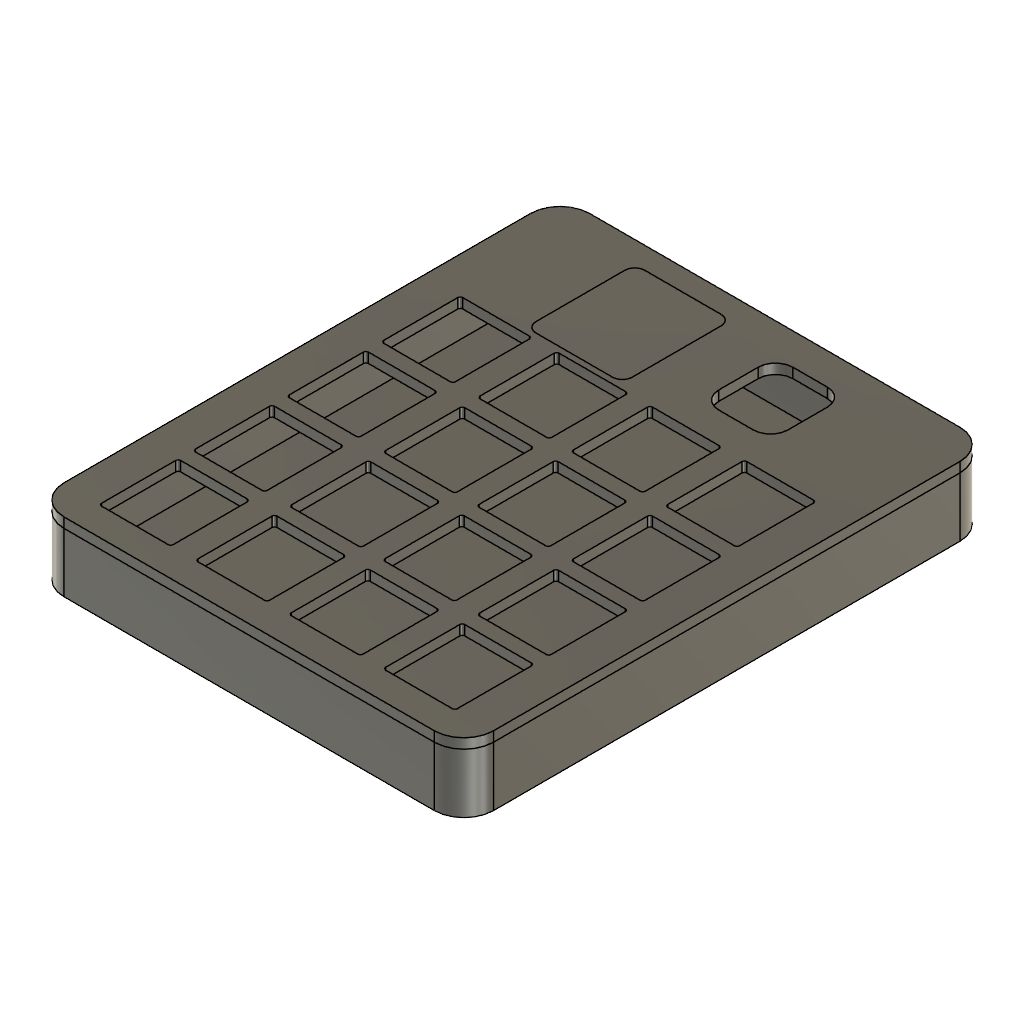
Untitled (Autodesk Fusion 360 design; units mm, degrees)
part number: 2026-09-21-00-24-33-049
Autodesk Fusion 360 part; units mm, degrees
sketch "Sketch2" plane through (0, 0, 0) normal (0, 0, 1) x (1, 0, 0)
sketch "Sketch3" plane through (0, 0, 0) normal (0, 0, 1) x (1, 0, 0)
  line L0 (0, 0) -> (80.94, 0)
  line L1 (80.94, 0) -> (80.94, 100.4)
  line L2 (80.94, 100.4) -> (0, 100.4)
  line L3 (0, 100.4) -> (0, 0)
  line L4 (3, 103.4) -> (77.94, 103.4)
  line L5 (83.94, 97.4) -> (83.94, 3)
  line L6 (77.94, -3) -> (3, -3)
  line L7 (-3, 3) -> (-3, 97.4)
  arc A0 (77.94, -3) -> (83.94, 3) centre (77.94, 3) ccw
  arc A1 (83.94, 97.4) -> (77.94, 103.4) centre (77.94, 97.4) ccw
  arc A2 (3, 103.4) -> (-3, 97.4) centre (3, 97.4) ccw
  arc A3 (-3, 3) -> (3, -3) centre (3, 3) ccw
  point P0 (82.94, -2)
  point P1 (-2, -2)
  point P2 (-3, 103.4)
  point P3 (83.94, 103.4)
  dimension "d5" = 80.94
  dimension "d6" = 100.4
  dimension "d26" = 86.94
  dimension "d27" = 6
  constraint horizontal L0
  constraint vertical L1
  constraint horizontal L2
  constraint vertical L3
  constraint coincident L0.start L3.end
  constraint perpendicular L1 L4
  constraint perpendicular L0 L5
  constraint perpendicular L5 L6
  constraint perpendicular L4 L7
  constraint tangent L5 A0
  constraint tangent L6 A0
  constraint coincident P3 L4
  constraint coincident P3 L5
  constraint tangent L4 A1
  constraint tangent L5 A1
  constraint equal A0 A1
  constraint coincident P2 L4
  constraint coincident P2 L7
  constraint tangent L4 A2
  constraint tangent L7 A2
  constraint equal A0 A2
  constraint tangent L6 A3
  constraint tangent L7 A3
  constraint equal A0 A3
  measures "d5" distance of L0.start L0.end
  measures "d6" distance of L0.start L2.end
  measures "d26" distance of P2 P3
  measures "d27" radius of A0
extrude "Extrude9" add sketch "Sketch3" along normal blind 2 contours L0 L1 L2 L3 | L4 L5 L6 L7 A0 A1 A2 A3 makes body 1
extrude "Extrude10" add sketch "Sketch3" along normal blind 12 bodies 1
sketch "Sketch4" plane through (0, 0, 12) normal (0, 0, 1) x (-1, 0, 0)
  line L0 (0, 0) -> (0, -100.4)
  line L1 (0, -100.4) -> (-80.94, -100.4)
  line L2 (-80.94, -100.4) -> (-80.94, 0)
  line L3 (-80.94, 0) -> (0, 0)
  arc A0 (-3, -103.4) -> (3, -97.4) centre (-3, -97.4) ccw
  line L4 (3, -97.4) -> (3, -3)
  arc A1 (3, -3) -> (-3, 3) centre (-3, -3) ccw
  line L5 (-3, 3) -> (-77.94, 3)
  arc A2 (-77.94, 3) -> (-83.94, -3) centre (-77.94, -3) ccw
  line L6 (-83.94, -3) -> (-83.94, -97.4)
  arc A3 (-83.94, -97.4) -> (-77.94, -103.4) centre (-77.94, -97.4) ccw
  line L7 (-77.94, -103.4) -> (-3, -103.4)
  line L8 (0, 0) -> (-80.94, 0)
  line L9 (-80.94, 0) -> (-80.94, -100.4)
  line L10 (-80.94, -100.4) -> (0, -100.4)
  line L11 (0, -100.4) -> (0, 0)
  line L12 (-4.9, -75.8) -> (-18.4, -75.8)
  line L13 (-18.9, -75.3) -> (-18.9, -60.3)
  line L14 (-18.4, -59.8) -> (-4.9, -59.8)
  line L15 (-4.4, -60.3) -> (-4.4, -75.3)
  line L16 (-38.4, -75.3) -> (-38.4, -60.3)
  line L17 (-37.9, -59.8) -> (-24.4, -59.8)
  line L18 (-23.9, -60.3) -> (-23.9, -75.3)
  line L19 (-24.4, -75.8) -> (-37.9, -75.8)
  line L20 (-57.3, -75.3) -> (-57.3, -60.3)
  line L21 (-56.8, -59.8) -> (-43.3, -59.8)
  line L22 (-42.8, -60.3) -> (-42.8, -75.3)
  line L23 (-43.3, -75.8) -> (-56.8, -75.8)
  line L24 (-76.4, -75.3) -> (-76.4, -60.3)
  line L25 (-75.9, -59.8) -> (-62.4, -59.8)
  line L26 (-61.9, -60.3) -> (-61.9, -75.3)
  line L27 (-62.4, -75.8) -> (-75.9, -75.8)
  line L28 (-4.4, -41.2) -> (-4.4, -56.2)
  line L29 (-18.4, -40.7) -> (-4.9, -40.7)
  line L30 (-18.9, -56.2) -> (-18.9, -41.2)
  line L31 (-4.9, -56.7) -> (-18.4, -56.7)
  line L32 (-23.9, -41.2) -> (-23.9, -56.2)
  line L33 (-24.4, -56.7) -> (-37.9, -56.7)
  line L34 (-38.4, -56.2) -> (-38.4, -41.2)
  line L35 (-37.9, -40.7) -> (-24.4, -40.7)
  line L36 (-42.8, -41.2) -> (-42.8, -56.2)
  line L37 (-56.8, -40.7) -> (-43.3, -40.7)
  line L38 (-57.3, -56.2) -> (-57.3, -41.2)
  line L39 (-43.3, -56.7) -> (-56.8, -56.7)
  line L40 (-62.4, -56.7) -> (-75.9, -56.7)
  line L41 (-61.9, -41.2) -> (-61.9, -56.2)
  line L42 (-75.9, -40.7) -> (-62.4, -40.7)
  line L43 (-76.4, -56.2) -> (-76.4, -41.2)
  line L44 (-4.4, -22.2) -> (-4.4, -37.2)
  line L45 (-18.4, -21.7) -> (-4.9, -21.7)
  line L46 (-18.9, -37.2) -> (-18.9, -22.2)
  line L47 (-4.9, -37.7) -> (-18.4, -37.7)
  line L48 (-23.9, -22.2) -> (-23.9, -37.2)
  line L49 (-24.4, -37.7) -> (-37.9, -37.7)
  line L50 (-38.4, -37.2) -> (-38.4, -22.2)
  line L51 (-37.9, -21.7) -> (-24.4, -21.7)
  line L52 (-42.8, -22.2) -> (-42.8, -37.2)
  line L53 (-56.8, -21.7) -> (-43.3, -21.7)
  line L54 (-57.3, -37.2) -> (-57.3, -22.2)
  line L55 (-43.3, -37.7) -> (-56.8, -37.7)
  line L56 (-62.4, -37.7) -> (-75.9, -37.7)
  line L57 (-61.9, -22.2) -> (-61.9, -37.2)
  line L58 (-75.9, -21.7) -> (-62.4, -21.7)
  line L59 (-76.4, -37.2) -> (-76.4, -22.2)
  line L60 (-4.4, -3.2) -> (-4.4, -18.2)
  line L61 (-18.4, -2.7) -> (-4.9, -2.7)
  line L62 (-18.9, -18.2) -> (-18.9, -3.2)
  line L63 (-4.9, -18.7) -> (-18.4, -18.7)
  line L64 (-23.9, -3.2) -> (-23.9, -18.2)
  line L65 (-24.4, -18.7) -> (-37.9, -18.7)
  line L66 (-38.4, -18.2) -> (-38.4, -3.2)
  line L67 (-37.9, -2.7) -> (-24.4, -2.7)
  line L68 (-42.8, -3.2) -> (-42.8, -18.2)
  line L69 (-56.8, -2.7) -> (-43.3, -2.7)
  line L70 (-57.3, -18.2) -> (-57.3, -3.2)
  line L71 (-43.3, -18.7) -> (-56.8, -18.7)
  line L72 (-62.4, -18.7) -> (-75.9, -18.7)
  line L73 (-61.9, -3.2) -> (-61.9, -18.2)
  line L74 (-75.9, -2.7) -> (-62.4, -2.7)
  line L75 (-76.4, -18.2) -> (-76.4, -3.2)
  line L76 (-50.5, -97) -> (-57.5, -97)
  line L77 (-61, -93.5) -> (-61, -85.5)
  line L78 (-57.5, -82) -> (-50.5, -82)
  line L79 (-47, -85.5) -> (-47, -93.5)
  arc A4 (-18.9, -75.3) -> (-18.4, -75.8) centre (-18.4, -75.3) ccw
  arc A5 (-18.4, -59.8) -> (-18.9, -60.3) centre (-18.4, -60.3) ccw
  arc A6 (-4.4, -60.3) -> (-4.9, -59.8) centre (-4.9, -60.3) ccw
  arc A7 (-4.9, -75.8) -> (-4.4, -75.3) centre (-4.9, -75.3) ccw
  arc A8 (-24.4, -75.8) -> (-23.9, -75.3) centre (-24.4, -75.3) ccw
  arc A9 (-38.4, -75.3) -> (-37.9, -75.8) centre (-37.9, -75.3) ccw
  arc A10 (-37.9, -59.8) -> (-38.4, -60.3) centre (-37.9, -60.3) ccw
  arc A11 (-23.9, -60.3) -> (-24.4, -59.8) centre (-24.4, -60.3) ccw
  arc A12 (-42.8, -60.3) -> (-43.3, -59.8) centre (-43.3, -60.3) ccw
  arc A13 (-56.8, -59.8) -> (-57.3, -60.3) centre (-56.8, -60.3) ccw
  arc A14 (-57.3, -75.3) -> (-56.8, -75.8) centre (-56.8, -75.3) ccw
  arc A15 (-43.3, -75.8) -> (-42.8, -75.3) centre (-43.3, -75.3) ccw
  arc A16 (-62.4, -75.8) -> (-61.9, -75.3) centre (-62.4, -75.3) ccw
  arc A17 (-61.9, -60.3) -> (-62.4, -59.8) centre (-62.4, -60.3) ccw
  arc A18 (-75.9, -59.8) -> (-76.4, -60.3) centre (-75.9, -60.3) ccw
  arc A19 (-76.4, -75.3) -> (-75.9, -75.8) centre (-75.9, -75.3) ccw
  arc A20 (-76.4, -56.2) -> (-75.9, -56.7) centre (-75.9, -56.2) ccw
  arc A21 (-75.9, -40.7) -> (-76.4, -41.2) centre (-75.9, -41.2) ccw
  arc A22 (-61.9, -41.2) -> (-62.4, -40.7) centre (-62.4, -41.2) ccw
  arc A23 (-62.4, -56.7) -> (-61.9, -56.2) centre (-62.4, -56.2) ccw
  arc A24 (-57.3, -56.2) -> (-56.8, -56.7) centre (-56.8, -56.2) ccw
  arc A25 (-43.3, -56.7) -> (-42.8, -56.2) centre (-43.3, -56.2) ccw
  arc A26 (-42.8, -41.2) -> (-43.3, -40.7) centre (-43.3, -41.2) ccw
  arc A27 (-56.8, -40.7) -> (-57.3, -41.2) centre (-56.8, -41.2) ccw
  arc A28 (-37.9, -40.7) -> (-38.4, -41.2) centre (-37.9, -41.2) ccw
  arc A29 (-38.4, -56.2) -> (-37.9, -56.7) centre (-37.9, -56.2) ccw
  arc A30 (-24.4, -56.7) -> (-23.9, -56.2) centre (-24.4, -56.2) ccw
  arc A31 (-23.9, -41.2) -> (-24.4, -40.7) centre (-24.4, -41.2) ccw
  arc A32 (-18.4, -40.7) -> (-18.9, -41.2) centre (-18.4, -41.2) ccw
  arc A33 (-18.9, -56.2) -> (-18.4, -56.7) centre (-18.4, -56.2) ccw
  arc A34 (-4.9, -56.7) -> (-4.4, -56.2) centre (-4.9, -56.2) ccw
  arc A35 (-4.4, -41.2) -> (-4.9, -40.7) centre (-4.9, -41.2) ccw
  arc A36 (-4.9, -37.7) -> (-4.4, -37.2) centre (-4.9, -37.2) ccw
  arc A37 (-4.4, -22.2) -> (-4.9, -21.7) centre (-4.9, -22.2) ccw
  arc A38 (-18.4, -21.7) -> (-18.9, -22.2) centre (-18.4, -22.2) ccw
  arc A39 (-18.9, -37.2) -> (-18.4, -37.7) centre (-18.4, -37.2) ccw
  arc A40 (-24.4, -37.7) -> (-23.9, -37.2) centre (-24.4, -37.2) ccw
  arc A41 (-23.9, -22.2) -> (-24.4, -21.7) centre (-24.4, -22.2) ccw
  arc A42 (-37.9, -21.7) -> (-38.4, -22.2) centre (-37.9, -22.2) ccw
  arc A43 (-38.4, -37.2) -> (-37.9, -37.7) centre (-37.9, -37.2) ccw
  arc A44 (-43.3, -37.7) -> (-42.8, -37.2) centre (-43.3, -37.2) ccw
  arc A45 (-42.8, -22.2) -> (-43.3, -21.7) centre (-43.3, -22.2) ccw
  arc A46 (-56.8, -21.7) -> (-57.3, -22.2) centre (-56.8, -22.2) ccw
  arc A47 (-57.3, -37.2) -> (-56.8, -37.7) centre (-56.8, -37.2) ccw
  arc A48 (-62.4, -37.7) -> (-61.9, -37.2) centre (-62.4, -37.2) ccw
  arc A49 (-61.9, -22.2) -> (-62.4, -21.7) centre (-62.4, -22.2) ccw
  arc A50 (-75.9, -21.7) -> (-76.4, -22.2) centre (-75.9, -22.2) ccw
  arc A51 (-76.4, -37.2) -> (-75.9, -37.7) centre (-75.9, -37.2) ccw
  arc A52 (-76.4, -18.2) -> (-75.9, -18.7) centre (-75.9, -18.2) ccw
  arc A53 (-62.4, -18.7) -> (-61.9, -18.2) centre (-62.4, -18.2) ccw
  arc A54 (-61.9, -3.2) -> (-62.4, -2.7) centre (-62.4, -3.2) ccw
  arc A55 (-75.9, -2.7) -> (-76.4, -3.2) centre (-75.9, -3.2) ccw
  arc A56 (-56.8, -2.7) -> (-57.3, -3.2) centre (-56.8, -3.2) ccw
  arc A57 (-57.3, -18.2) -> (-56.8, -18.7) centre (-56.8, -18.2) ccw
  arc A58 (-43.3, -18.7) -> (-42.8, -18.2) centre (-43.3, -18.2) ccw
  arc A59 (-42.8, -3.2) -> (-43.3, -2.7) centre (-43.3, -3.2) ccw
  arc A60 (-37.9, -2.7) -> (-38.4, -3.2) centre (-37.9, -3.2) ccw
  arc A61 (-38.4, -18.2) -> (-37.9, -18.7) centre (-37.9, -18.2) ccw
  arc A62 (-24.4, -18.7) -> (-23.9, -18.2) centre (-24.4, -18.2) ccw
  arc A63 (-23.9, -3.2) -> (-24.4, -2.7) centre (-24.4, -3.2) ccw
  arc A64 (-18.4, -2.7) -> (-18.9, -3.2) centre (-18.4, -3.2) ccw
  arc A65 (-18.9, -18.2) -> (-18.4, -18.7) centre (-18.4, -18.2) ccw
  arc A66 (-4.9, -18.7) -> (-4.4, -18.2) centre (-4.9, -18.2) ccw
  arc A67 (-4.4, -3.2) -> (-4.9, -2.7) centre (-4.9, -3.2) ccw
  arc A68 (-47, -85.5) -> (-50.5, -82) centre (-50.5, -85.5) ccw
  arc A69 (-57.5, -82) -> (-61, -85.5) centre (-57.5, -85.5) ccw
  arc A70 (-61, -93.5) -> (-57.5, -97) centre (-57.5, -93.5) ccw
  arc A71 (-50.5, -97) -> (-47, -93.5) centre (-50.5, -93.5) ccw
  dimension "d32" = 0.5
  dimension "d33" = 3.5
  constraint horizontal L8
  constraint vertical L9
  constraint horizontal L10
  constraint vertical L11
  constraint coincident L1.end L2.start
  constraint coincident L0.start L3.end
  constraint horizontal L12
  constraint vertical L13
  constraint horizontal L14
  constraint vertical L15
  constraint horizontal L19
  constraint vertical L16
  constraint horizontal L17
  constraint vertical L18
  constraint horizontal L23
  constraint vertical L20
  constraint horizontal L21
  constraint vertical L22
  constraint horizontal L27
  constraint vertical L24
  constraint horizontal L25
  constraint vertical L26
  constraint horizontal L31
  constraint vertical L30
  constraint horizontal L29
  constraint vertical L28
  constraint horizontal L33
  constraint vertical L34
  constraint horizontal L35
  constraint vertical L32
  constraint horizontal L39
  constraint vertical L38
  constraint horizontal L37
  constraint vertical L36
  constraint horizontal L40
  constraint vertical L43
  constraint horizontal L42
  constraint vertical L41
  constraint horizontal L47
  constraint vertical L46
  constraint horizontal L45
  constraint vertical L44
  constraint horizontal L49
  constraint vertical L50
  constraint horizontal L51
  constraint vertical L48
  constraint horizontal L55
  constraint vertical L54
  constraint horizontal L53
  constraint vertical L52
  constraint horizontal L56
  constraint vertical L59
  constraint horizontal L58
  constraint vertical L57
  constraint horizontal L63
  constraint vertical L62
  constraint horizontal L61
  constraint vertical L60
  constraint horizontal L65
  constraint vertical L66
  constraint horizontal L67
  constraint vertical L64
  constraint horizontal L71
  constraint vertical L70
  constraint horizontal L69
  constraint vertical L68
  constraint horizontal L72
  constraint vertical L75
  constraint horizontal L74
  constraint vertical L73
  constraint horizontal L76
  constraint vertical L77
  constraint horizontal L78
  constraint vertical L79
  constraint tangent L12 A4
  constraint tangent L13 A4
  constraint tangent L13 A5
  constraint tangent L14 A5
  constraint equal A4 A5
  constraint tangent L14 A6
  constraint tangent L15 A6
  constraint equal A4 A6
  constraint tangent L12 A7
  constraint tangent L15 A7
  constraint equal A4 A7
  constraint tangent L18 A8
  constraint tangent L19 A8
  constraint equal A4 A8
  constraint tangent L16 A9
  constraint tangent L19 A9
  constraint equal A4 A9
  constraint tangent L16 A10
  constraint tangent L17 A10
  constraint equal A4 A10
  constraint tangent L17 A11
  constraint tangent L18 A11
  constraint equal A4 A11
  constraint tangent L21 A12
  constraint tangent L22 A12
  constraint equal A4 A12
  constraint tangent L20 A13
  constraint tangent L21 A13
  constraint equal A4 A13
  constraint tangent L20 A14
  constraint tangent L23 A14
  constraint equal A4 A14
  constraint tangent L22 A15
  constraint tangent L23 A15
  constraint equal A4 A15
  constraint tangent L26 A16
  constraint tangent L27 A16
  constraint equal A4 A16
  constraint tangent L25 A17
  constraint tangent L26 A17
  constraint equal A4 A17
  constraint tangent L24 A18
  constraint tangent L25 A18
  constraint equal A4 A18
  constraint tangent L24 A19
  constraint tangent L27 A19
  constraint equal A4 A19
  constraint tangent L40 A20
  constraint tangent L43 A20
  constraint equal A4 A20
  constraint tangent L42 A21
  constraint tangent L43 A21
  constraint equal A4 A21
  constraint tangent L41 A22
  constraint tangent L42 A22
  constraint equal A4 A22
  constraint tangent L40 A23
  constraint tangent L41 A23
  constraint equal A4 A23
  constraint tangent L38 A24
  constraint tangent L39 A24
  constraint equal A4 A24
  constraint tangent L36 A25
  constraint tangent L39 A25
  constraint equal A4 A25
  constraint tangent L36 A26
  constraint tangent L37 A26
  constraint equal A4 A26
  constraint tangent L37 A27
  constraint tangent L38 A27
  constraint equal A4 A27
  constraint tangent L34 A28
  constraint tangent L35 A28
  constraint equal A4 A28
  constraint tangent L33 A29
  constraint tangent L34 A29
  constraint equal A4 A29
  constraint tangent L32 A30
  constraint tangent L33 A30
  constraint equal A4 A30
  constraint tangent L32 A31
  constraint tangent L35 A31
  constraint equal A4 A31
  constraint tangent L29 A32
  constraint tangent L30 A32
  constraint equal A4 A32
  constraint tangent L30 A33
  constraint tangent L31 A33
  constraint equal A4 A33
  constraint tangent L28 A34
  constraint tangent L31 A34
  constraint equal A4 A34
  constraint tangent L28 A35
  constraint tangent L29 A35
  constraint equal A4 A35
  constraint tangent L44 A36
  constraint tangent L47 A36
  constraint equal A4 A36
  constraint tangent L44 A37
  constraint tangent L45 A37
  constraint equal A4 A37
  constraint tangent L45 A38
  constraint tangent L46 A38
  constraint equal A4 A38
  constraint tangent L46 A39
  constraint tangent L47 A39
  constraint equal A4 A39
  constraint tangent L48 A40
  constraint tangent L49 A40
  constraint equal A4 A40
  constraint tangent L48 A41
  constraint tangent L51 A41
  constraint equal A4 A41
  constraint tangent L50 A42
  constraint tangent L51 A42
  constraint equal A4 A42
  constraint tangent L49 A43
  constraint tangent L50 A43
  constraint equal A4 A43
  constraint tangent L52 A44
  constraint tangent L55 A44
  constraint equal A4 A44
  constraint tangent L52 A45
  constraint tangent L53 A45
  constraint equal A4 A45
  constraint tangent L53 A46
  constraint tangent L54 A46
  constraint equal A4 A46
  constraint tangent L54 A47
  constraint tangent L55 A47
  constraint equal A4 A47
  constraint tangent L56 A48
  constraint tangent L57 A48
  constraint equal A4 A48
  constraint tangent L57 A49
  constraint tangent L58 A49
  constraint equal A4 A49
  constraint tangent L58 A50
  constraint tangent L59 A50
  constraint equal A4 A50
  constraint tangent L56 A51
  constraint tangent L59 A51
  constraint equal A4 A51
  constraint tangent L72 A52
  constraint tangent L75 A52
  constraint equal A4 A52
  constraint tangent L72 A53
  constraint tangent L73 A53
  constraint equal A4 A53
  constraint tangent L73 A54
  constraint tangent L74 A54
  constraint equal A4 A54
  constraint tangent L74 A55
  constraint tangent L75 A55
  constraint equal A4 A55
  constraint tangent L69 A56
  constraint tangent L70 A56
  constraint equal A4 A56
  constraint tangent L70 A57
  constraint tangent L71 A57
  constraint equal A4 A57
  constraint tangent L68 A58
  constraint tangent L71 A58
  constraint equal A4 A58
  constraint tangent L68 A59
  constraint tangent L69 A59
  constraint equal A4 A59
  constraint tangent L66 A60
  constraint tangent L67 A60
  constraint equal A4 A60
  constraint tangent L65 A61
  constraint tangent L66 A61
  constraint equal A4 A61
  constraint tangent L64 A62
  constraint tangent L65 A62
  constraint equal A4 A62
  constraint tangent L64 A63
  constraint tangent L67 A63
  constraint equal A4 A63
  constraint tangent L61 A64
  constraint tangent L62 A64
  constraint equal A4 A64
  constraint tangent L62 A65
  constraint tangent L63 A65
  constraint equal A4 A65
  constraint tangent L60 A66
  constraint tangent L63 A66
  constraint equal A4 A66
  constraint tangent L60 A67
  constraint tangent L61 A67
  constraint equal A4 A67
  constraint tangent L78 A68
  constraint tangent L79 A68
  constraint tangent L77 A69
  constraint tangent L78 A69
  constraint equal A68 A69
  constraint tangent L76 A70
  constraint tangent L77 A70
  constraint equal A68 A70
  constraint tangent L76 A71
  constraint tangent L79 A71
  constraint equal A68 A71
  measures "d32" radius of A4
  measures "d33" radius of A68
extrude "Extrude11" add sketch "Sketch4" along normal blind 2 separate body contours L0 L1 L2 L3 L8 L9 L10 L11 makes body 2
extrude "Extrude12" add sketch "Sketch3" along normal blind 2 separate body makes body 3
move_body "Move1" bodies 3 to x (1, 0, 0) y (0, 1, 0) z (0, 0, 1) at (0, 0, 12)
combine "Combine1" operation add target body 3 tool bodies 2
sketch "Sketch5" plane through (0, 0, 14) normal (0, 0, 1) x (-1, 0, 0)
  arc A0 (-61, -93.5) -> (-57.5, -97) centre (-57.5, -93.5) ccw
  line L0 (-61, -93.5) -> (-61, -85.5)
  arc A1 (-57.5, -82) -> (-61, -85.5) centre (-57.5, -85.5) ccw
  line L1 (-57.5, -82) -> (-50.5, -82)
  arc A2 (-47, -85.5) -> (-50.5, -82) centre (-50.5, -85.5) ccw
  line L2 (-47, -85.5) -> (-47, -93.5)
  arc A3 (-50.5, -97) -> (-47, -93.5) centre (-50.5, -93.5) ccw
  line L3 (-50.5, -97) -> (-57.5, -97)
  arc A4 (-75.9, -21.7) -> (-76.4, -22.2) centre (-75.9, -22.2) ccw
  line L4 (-75.9, -21.7) -> (-62.4, -21.7)
  arc A5 (-61.9, -22.2) -> (-62.4, -21.7) centre (-62.4, -22.2) ccw
  line L5 (-61.9, -22.2) -> (-61.9, -37.2)
  arc A6 (-62.4, -37.7) -> (-61.9, -37.2) centre (-62.4, -37.2) ccw
  line L6 (-62.4, -37.7) -> (-75.9, -37.7)
  arc A7 (-76.4, -37.2) -> (-75.9, -37.7) centre (-75.9, -37.2) ccw
  line L7 (-76.4, -37.2) -> (-76.4, -22.2)
  arc A8 (-61.9, -3.2) -> (-62.4, -2.7) centre (-62.4, -3.2) ccw
  line L8 (-61.9, -3.2) -> (-61.9, -18.2)
  arc A9 (-62.4, -18.7) -> (-61.9, -18.2) centre (-62.4, -18.2) ccw
  line L9 (-62.4, -18.7) -> (-75.9, -18.7)
  arc A10 (-76.4, -18.2) -> (-75.9, -18.7) centre (-75.9, -18.2) ccw
  line L10 (-76.4, -18.2) -> (-76.4, -3.2)
  arc A11 (-75.9, -2.7) -> (-76.4, -3.2) centre (-75.9, -3.2) ccw
  line L11 (-75.9, -2.7) -> (-62.4, -2.7)
  arc A12 (-18.4, -21.7) -> (-18.9, -22.2) centre (-18.4, -22.2) ccw
  line L12 (-18.4, -21.7) -> (-4.9, -21.7)
  arc A13 (-4.4, -22.2) -> (-4.9, -21.7) centre (-4.9, -22.2) ccw
  line L13 (-4.4, -22.2) -> (-4.4, -37.2)
  arc A14 (-4.9, -37.7) -> (-4.4, -37.2) centre (-4.9, -37.2) ccw
  line L14 (-4.9, -37.7) -> (-18.4, -37.7)
  arc A15 (-18.9, -37.2) -> (-18.4, -37.7) centre (-18.4, -37.2) ccw
  line L15 (-18.9, -37.2) -> (-18.9, -22.2)
  arc A16 (-24.4, -18.7) -> (-23.9, -18.2) centre (-24.4, -18.2) ccw
  line L16 (-24.4, -18.7) -> (-37.9, -18.7)
  arc A17 (-38.4, -18.2) -> (-37.9, -18.7) centre (-37.9, -18.2) ccw
  line L17 (-38.4, -18.2) -> (-38.4, -3.2)
  arc A18 (-37.9, -2.7) -> (-38.4, -3.2) centre (-37.9, -3.2) ccw
  line L18 (-37.9, -2.7) -> (-24.4, -2.7)
  arc A19 (-23.9, -3.2) -> (-24.4, -2.7) centre (-24.4, -3.2) ccw
  line L19 (-23.9, -3.2) -> (-23.9, -18.2)
  arc A20 (-18.9, -75.3) -> (-18.4, -75.8) centre (-18.4, -75.3) ccw
  line L20 (-18.9, -75.3) -> (-18.9, -60.3)
  arc A21 (-18.4, -59.8) -> (-18.9, -60.3) centre (-18.4, -60.3) ccw
  line L21 (-18.4, -59.8) -> (-4.9, -59.8)
  arc A22 (-4.4, -60.3) -> (-4.9, -59.8) centre (-4.9, -60.3) ccw
  line L22 (-4.4, -60.3) -> (-4.4, -75.3)
  arc A23 (-4.9, -75.8) -> (-4.4, -75.3) centre (-4.9, -75.3) ccw
  line L23 (-4.9, -75.8) -> (-18.4, -75.8)
  arc A24 (-4.9, -56.7) -> (-4.4, -56.2) centre (-4.9, -56.2) ccw
  line L24 (-4.9, -56.7) -> (-18.4, -56.7)
  arc A25 (-18.9, -56.2) -> (-18.4, -56.7) centre (-18.4, -56.2) ccw
  line L25 (-18.9, -56.2) -> (-18.9, -41.2)
  arc A26 (-18.4, -40.7) -> (-18.9, -41.2) centre (-18.4, -41.2) ccw
  line L26 (-18.4, -40.7) -> (-4.9, -40.7)
  arc A27 (-4.4, -41.2) -> (-4.9, -40.7) centre (-4.9, -41.2) ccw
  line L27 (-4.4, -41.2) -> (-4.4, -56.2)
  arc A28 (-75.9, -59.8) -> (-76.4, -60.3) centre (-75.9, -60.3) ccw
  line L28 (-75.9, -59.8) -> (-62.4, -59.8)
  arc A29 (-61.9, -60.3) -> (-62.4, -59.8) centre (-62.4, -60.3) ccw
  line L29 (-61.9, -60.3) -> (-61.9, -75.3)
  arc A30 (-62.4, -75.8) -> (-61.9, -75.3) centre (-62.4, -75.3) ccw
  line L30 (-62.4, -75.8) -> (-75.9, -75.8)
  arc A31 (-76.4, -75.3) -> (-75.9, -75.8) centre (-75.9, -75.3) ccw
  line L31 (-76.4, -75.3) -> (-76.4, -60.3)
  arc A32 (-4.9, -18.7) -> (-4.4, -18.2) centre (-4.9, -18.2) ccw
  line L32 (-4.9, -18.7) -> (-18.4, -18.7)
  arc A33 (-18.9, -18.2) -> (-18.4, -18.7) centre (-18.4, -18.2) ccw
  line L33 (-18.9, -18.2) -> (-18.9, -3.2)
  arc A34 (-18.4, -2.7) -> (-18.9, -3.2) centre (-18.4, -3.2) ccw
  line L34 (-18.4, -2.7) -> (-4.9, -2.7)
  arc A35 (-4.4, -3.2) -> (-4.9, -2.7) centre (-4.9, -3.2) ccw
  line L35 (-4.4, -3.2) -> (-4.4, -18.2)
  arc A36 (-42.8, -41.2) -> (-43.3, -40.7) centre (-43.3, -41.2) ccw
  line L36 (-42.8, -41.2) -> (-42.8, -56.2)
  arc A37 (-43.3, -56.7) -> (-42.8, -56.2) centre (-43.3, -56.2) ccw
  line L37 (-43.3, -56.7) -> (-56.8, -56.7)
  arc A38 (-57.3, -56.2) -> (-56.8, -56.7) centre (-56.8, -56.2) ccw
  line L38 (-57.3, -56.2) -> (-57.3, -41.2)
  arc A39 (-56.8, -40.7) -> (-57.3, -41.2) centre (-56.8, -41.2) ccw
  line L39 (-56.8, -40.7) -> (-43.3, -40.7)
  arc A40 (-37.9, -21.7) -> (-38.4, -22.2) centre (-37.9, -22.2) ccw
  line L40 (-37.9, -21.7) -> (-24.4, -21.7)
  arc A41 (-23.9, -22.2) -> (-24.4, -21.7) centre (-24.4, -22.2) ccw
  line L41 (-23.9, -22.2) -> (-23.9, -37.2)
  arc A42 (-24.4, -37.7) -> (-23.9, -37.2) centre (-24.4, -37.2) ccw
  line L42 (-24.4, -37.7) -> (-37.9, -37.7)
  arc A43 (-38.4, -37.2) -> (-37.9, -37.7) centre (-37.9, -37.2) ccw
  line L43 (-38.4, -37.2) -> (-38.4, -22.2)
  arc A44 (-76.4, -56.2) -> (-75.9, -56.7) centre (-75.9, -56.2) ccw
  line L44 (-76.4, -56.2) -> (-76.4, -41.2)
  arc A45 (-75.9, -40.7) -> (-76.4, -41.2) centre (-75.9, -41.2) ccw
  line L45 (-75.9, -40.7) -> (-62.4, -40.7)
  arc A46 (-61.9, -41.2) -> (-62.4, -40.7) centre (-62.4, -41.2) ccw
  line L46 (-61.9, -41.2) -> (-61.9, -56.2)
  arc A47 (-62.4, -56.7) -> (-61.9, -56.2) centre (-62.4, -56.2) ccw
  line L47 (-62.4, -56.7) -> (-75.9, -56.7)
  arc A48 (-24.4, -56.7) -> (-23.9, -56.2) centre (-24.4, -56.2) ccw
  line L48 (-24.4, -56.7) -> (-37.9, -56.7)
  arc A49 (-38.4, -56.2) -> (-37.9, -56.7) centre (-37.9, -56.2) ccw
  line L49 (-38.4, -56.2) -> (-38.4, -41.2)
  arc A50 (-37.9, -40.7) -> (-38.4, -41.2) centre (-37.9, -41.2) ccw
  line L50 (-37.9, -40.7) -> (-24.4, -40.7)
  arc A51 (-23.9, -41.2) -> (-24.4, -40.7) centre (-24.4, -41.2) ccw
  line L51 (-23.9, -41.2) -> (-23.9, -56.2)
  arc A52 (-57.3, -75.3) -> (-56.8, -75.8) centre (-56.8, -75.3) ccw
  line L52 (-57.3, -75.3) -> (-57.3, -60.3)
  arc A53 (-56.8, -59.8) -> (-57.3, -60.3) centre (-56.8, -60.3) ccw
  line L53 (-56.8, -59.8) -> (-43.3, -59.8)
  arc A54 (-42.8, -60.3) -> (-43.3, -59.8) centre (-43.3, -60.3) ccw
  line L54 (-42.8, -60.3) -> (-42.8, -75.3)
  arc A55 (-43.3, -75.8) -> (-42.8, -75.3) centre (-43.3, -75.3) ccw
  line L55 (-43.3, -75.8) -> (-56.8, -75.8)
  arc A56 (-43.3, -18.7) -> (-42.8, -18.2) centre (-43.3, -18.2) ccw
  line L56 (-43.3, -18.7) -> (-56.8, -18.7)
  arc A57 (-57.3, -18.2) -> (-56.8, -18.7) centre (-56.8, -18.2) ccw
  line L57 (-57.3, -18.2) -> (-57.3, -3.2)
  arc A58 (-56.8, -2.7) -> (-57.3, -3.2) centre (-56.8, -3.2) ccw
  line L58 (-56.8, -2.7) -> (-43.3, -2.7)
  arc A59 (-42.8, -3.2) -> (-43.3, -2.7) centre (-43.3, -3.2) ccw
  line L59 (-42.8, -3.2) -> (-42.8, -18.2)
  arc A60 (-24.4, -75.8) -> (-23.9, -75.3) centre (-24.4, -75.3) ccw
  line L60 (-24.4, -75.8) -> (-37.9, -75.8)
  arc A61 (-38.4, -75.3) -> (-37.9, -75.8) centre (-37.9, -75.3) ccw
  line L61 (-38.4, -75.3) -> (-38.4, -60.3)
  arc A62 (-37.9, -59.8) -> (-38.4, -60.3) centre (-37.9, -60.3) ccw
  line L62 (-37.9, -59.8) -> (-24.4, -59.8)
  arc A63 (-23.9, -60.3) -> (-24.4, -59.8) centre (-24.4, -60.3) ccw
  line L63 (-23.9, -60.3) -> (-23.9, -75.3)
  arc A64 (-56.8, -21.7) -> (-57.3, -22.2) centre (-56.8, -22.2) ccw
  line L64 (-56.8, -21.7) -> (-43.3, -21.7)
  arc A65 (-42.8, -22.2) -> (-43.3, -21.7) centre (-43.3, -22.2) ccw
  line L65 (-42.8, -22.2) -> (-42.8, -37.2)
  arc A66 (-43.3, -37.7) -> (-42.8, -37.2) centre (-43.3, -37.2) ccw
  line L66 (-43.3, -37.7) -> (-56.8, -37.7)
  arc A67 (-57.3, -37.2) -> (-56.8, -37.7) centre (-56.8, -37.2) ccw
  line L67 (-57.3, -37.2) -> (-57.3, -22.2)
  arc A68 (-3, -103.4) -> (3, -97.4) centre (-3, -97.4) ccw
  line L68 (3, -97.4) -> (3, -3)
  arc A69 (3, -3) -> (-3, 3) centre (-3, -3) ccw
  line L69 (-3, 3) -> (-77.94, 3)
  arc A70 (-77.94, 3) -> (-83.94, -3) centre (-77.94, -3) ccw
  line L70 (-83.94, -3) -> (-83.94, -97.4)
  arc A71 (-83.94, -97.4) -> (-77.94, -103.4) centre (-77.94, -97.4) ccw
  line L71 (-77.94, -103.4) -> (-3, -103.4)
  line L72 (-18.5166, -99) -> (-34, -99)
  line L73 (-36, -97) -> (-36, -79)
  line L74 (-34, -77) -> (-18.5166, -77)
  line L75 (-16.5166, -79) -> (-16.5166, -97)
  arc A72 (-18.5166, -99) -> (-16.5166, -97) centre (-18.5166, -97) ccw
  arc A73 (-36, -97) -> (-34, -99) centre (-34, -97) ccw
  arc A74 (-34, -77) -> (-36, -79) centre (-34, -79) ccw
  arc A75 (-16.5166, -79) -> (-18.5166, -77) centre (-18.5166, -79) ccw
  dimension "d38" = 2
  constraint horizontal L72
  constraint vertical L73
  constraint horizontal L74
  constraint vertical L75
  constraint tangent L72 A72
  constraint tangent L75 A72
  constraint tangent L72 A73
  constraint tangent L73 A73
  constraint equal A72 A73
  constraint tangent L73 A74
  constraint tangent L74 A74
  constraint equal A72 A74
  constraint tangent L74 A75
  constraint tangent L75 A75
  constraint equal A72 A75
  measures "d38" radius of A72
extrude "Extrude13" cut sketch "Sketch5" against normal blind 2 contours L72 L73 L74 L75 A72 A73 A74 A75 bodies 3
extrude "Extrude14" add sketch "Sketch5" against normal blind 2 separate body contours L72 L73 L74 L75 A72 A73 A74 A75 makes body 4
sketch "Sketch6" plane through (0, 103.4, 0) normal (0, 1, 0) x (-1, 0, 0)
  line L0 (-77.94, 0) -> (-3, 0)
  line L1 (-3, 0) -> (-3, 12)
  line L2 (-3, 12) -> (-77.94, 12)
  line L3 (-77.94, 12) -> (-77.94, 0)
  line L4 (-22.0085, 5.3541) -> (-30.4097, 5.3541)
  line L5 (-30.9097, 5.8541) -> (-30.9097, 8.4904)
  line L6 (-30.4097, 8.9904) -> (-22.0085, 8.9904)
  line L7 (-21.5085, 8.4904) -> (-21.5085, 5.8541)
  arc A0 (-30.4097, 8.9904) -> (-30.9097, 8.4904) centre (-30.4097, 8.4904) ccw
  arc A1 (-21.5085, 8.4904) -> (-22.0085, 8.9904) centre (-22.0085, 8.4904) ccw
  arc A2 (-22.0085, 5.3541) -> (-21.5085, 5.8541) centre (-22.0085, 5.8541) ccw
  arc A3 (-30.9097, 5.8541) -> (-30.4097, 5.3541) centre (-30.4097, 5.8541) ccw
  dimension "d43" = 0.5
  constraint horizontal L4
  constraint vertical L5
  constraint horizontal L6
  constraint vertical L7
  constraint tangent L5 A0
  constraint tangent L6 A0
  constraint tangent L6 A1
  constraint tangent L7 A1
  constraint equal A0 A1
  constraint tangent L4 A2
  constraint tangent L7 A2
  constraint equal A0 A2
  constraint tangent L4 A3
  constraint tangent L5 A3
  constraint equal A0 A3
  measures "d43" radius of A0
extrude "Extrude15" cut sketch "Sketch6" against normal blind 4 contours L4 L5 L6 L7 A0 A1 A2 A3 bodies 1
equation "d26 = 80.940 mm + 6 mm"
